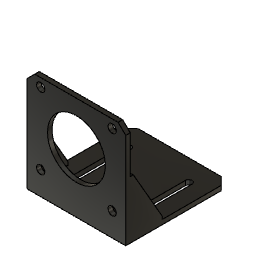
NEMA23 bracket (Autodesk Fusion 360 design; units mm, degrees)
Autodesk Fusion 360 part; units mm, degrees
note: some values were not read from the file. Set by a fixed rule: which sketch regions a step uses.
sketch "NEMA23 bracket front" plane through (0, 0, 0) normal (0, 1, 0) x (1, 0, 0)
  line L0 (-32.5, -3) -> (-32.5, -63)
  line L1 (-32.5, 0) -> (-32.5, -3)
  line L2 (32.5, 0) -> (-32.5, 0)
  line L3 (32.5, -63) -> (32.5, -3)
  line L4 (-32.5, -3) -> (32.5, -3)
  line L5 (-27.5, -68) -> (27.5, -68)
  line L6 (23.55, -15.45) -> (-23.55, -15.45) construction
  line L7 (32.5, -3) -> (32.5, 0)
  circle A0 centre (-23.55, -62.55) radius 2.75
  line L8 (32.5, 0) -> (32.5, -68) construction
  line L9 (23.55, -62.55) -> (-23.55, -62.55) construction
  circle A1 centre (23.55, -15.45) radius 2.75
  line L10 (32.5, -3) -> (-32.5, -3)
  circle A2 centre (0, -39) radius 19.05
  line L11 (-23.55, -62.55) -> (-23.55, -15.45) construction
  line L12 (23.55, -15.45) -> (23.55, -62.55) construction
  circle A3 centre (-23.55, -15.45) radius 2.75
  circle A4 centre (23.55, -62.55) radius 2.75
  line L13 (-32.5, -63) -> (-27.5, -68)
  line L14 (27.5, -68) -> (32.5, -63)
  dimension "d22" = 38.1
  dimension "d23" = 39
  dimension "d24" = 5.5
  dimension "d27" = 47.1
  dimension "d28" = 47.1
  dimension "d29" = 47.1
  dimension "d30" = 5.5
  dimension "d31" = 5.5
  dimension "d32" = 5.5
  dimension "d33" = 68
  dimension "d34" = 32.5
  dimension "d35" = 65
  dimension "d36" = 3
  dimension "d37" = 65
  dimension "d39" = 5.45
  dimension "d46" = 5
  dimension "d47" = 5
  constraint coincident L6.start A1.centre
  constraint perpendicular L6 L12
  constraint perpendicular L9 L12
  constraint coincident L9.start L12.end
  constraint coincident A0.centre L9.end
  constraint coincident L6.end L11.end
  constraint coincident L8 L3.start
  measures "d22" diameter of A2
  measures "d23" distance of A2.centre origin
  measures "d24" diameter of A1
  measures "d27" distance of L6.end L6.start
  measures "d28" distance of L6.start L9.start
  measures "d29" distance of A0.centre L9.start
  measures "d30" diameter of A4
  measures "d31" diameter of A0
  measures "d32" diameter of A3
  measures "d33" distance of L2.start L8.end
  measures "d34" distance of L2.start origin
  measures "d35" distance of L1.start L2.start
  measures "d36" distance of L2.start L3.end
  measures "d37" distance of L3.end L0.start
  measures "d39" distance of L9.start L5
  measures "d46" distance of L8.end L5.end
  measures "d47" distance of L8.end L3.start
extrude "Extrude1" add sketch "NEMA23 bracket front" along normal blind 68 contours L1 L2 L4 L7 L10 makes body 1
extrude "Extrude2" add sketch "NEMA23 bracket front" along normal blind 3 contours L0 L3 L4 L5 L10 L13 L14 bodies 1
sketch "NEMA23 bracket side" plane through (0, 0, 0) normal (1, 0, 0) x (0, 1, 0)
  line L0 (3, 3) -> (24, 3)
  line L1 (24, 3) -> (24, 5)
  line L2 (24, 5) -> (5, 38)
  line L3 (5, 38) -> (3, 38)
  line L4 (3, 38) -> (3, 3)
  dimension "d52" = 21
  dimension "d53" = 35
  dimension "d54" = 2
  dimension "d55" = 2
  dimension "d56" = 3
  dimension "d57" = 3
  constraint horizontal L0
  constraint perpendicular L0 L1
  constraint perpendicular L1 L3
  constraint perpendicular L0 L4
  measures "d52" distance of L0.start L0.end
  measures "d53" distance of L0.start L3.end
  measures "d54" distance of L2.end L3.end
  measures "d55" distance of L0.end L1.end
  measures "d56" horizontal distance of origin L0.start
  measures "d57" vertical distance of origin L0.start
extrude "Extrude3" add sketch "NEMA23 bracket side" along normal mid plane 65 bodies 1
extrude "Extrude4" cut sketch "NEMA23 bracket side" along normal mid plane 59 bodies 1
sketch "NEMA23 bracket top" plane through (0, 0, 3) normal (0, 0, 1) x (-1, 0, 0)
  line L0 (32.5, -24) -> (29.5, -24)
  line L1 (29.5, -24) -> (29.5, -3)
  line L2 (29.5, -3) -> (-29.5, -3)
  line L3 (-29.5, -3) -> (-29.5, -24)
  line L4 (-29.5, -24) -> (-32.5, -24)
  line L5 (-32.5, -24) -> (-32.5, -68)
  line L6 (-32.5, -68) -> (32.5, -68)
  line L7 (32.5, -68) -> (32.5, -24)
  line L8 (20, -54) -> (-20, -54) construction
  line L9 (-20, -54) -> (-20, -13) construction
  line L10 (-20, -13) -> (20, -13) construction
  line L11 (20, -13) -> (20, -54) construction
  line L12 (32.5, -68) -> (27.5, -68)
  line L13 (32.5, -68) -> (32.5, -63)
  line L14 (27.5, -68) -> (32.5, -63)
  line L15 (-32.5, -68) -> (-27.5, -68)
  line L16 (-32.5, -68) -> (-32.5, -63)
  line L17 (-32.5, -63) -> (-27.5, -68)
  line L18 (22.15, -54) -> (22.15, -13)
  line L19 (17.85, -54) -> (17.85, -13)
  line L20 (-17.85, -54) -> (-17.85, -13)
  line L21 (-22.15, -54) -> (-22.15, -13)
  arc A0 (17.85, -54) -> (22.15, -54) centre (20, -54) ccw
  arc A1 (22.15, -13) -> (17.85, -13) centre (20, -13) ccw
  arc A2 (-17.85, -13) -> (-22.15, -13) centre (-20, -13) ccw
  arc A3 (-22.15, -54) -> (-17.85, -54) centre (-20, -54) ccw
  dimension "d62" = 40
  dimension "d63" = 41
  dimension "d64" = 13
  dimension "d65" = 4.3
  dimension "d66" = 4.3
  dimension "d67" = 4.3
  dimension "d68" = 4.3
  dimension "d69" = 5
  dimension "d70" = 5
  dimension "d71" = 5
  dimension "d72" = 5
  constraint horizontal L8
  constraint vertical L9
  constraint horizontal L10
  constraint vertical L11
  constraint coincident L8.start L11.end
  constraint coincident L8.end L9.start
  constraint coincident L10.end L11.start
  constraint coincident L9.end L10.start
  constraint coincident L6.end L7.start
  constraint perpendicular L7 L12
  constraint coincident L7 L13.end
  constraint coincident L5.end L6.start
  constraint coincident L6 L15.end
  constraint perpendicular L15 L16
  constraint tangent L18 A1
  constraint parallel L11 L18
  constraint coincident L8 L19.start
  constraint coincident L10 L19.end
  constraint coincident L8 L20.start
  constraint coincident L10 L20.end
  constraint tangent L21 A2
  constraint parallel L9 L21
  measures "d62" distance of L9 L11
  measures "d63" distance of L8 L10
  measures "d64" distance of origin L10
  measures "d65" diameter of A0
  measures "d66" diameter of A3
  measures "d67" diameter of A1
  measures "d68" diameter of A2
  measures "d69" distance of L6.end L12.end
  measures "d70" distance of L6.end L13.end
  measures "d71" distance of L5.end L15.end
  measures "d72" distance of L5.end L16.end
extrude "Extrude5" cut sketch "NEMA23 bracket top" against normal blind 5 contours L18 L19 A0 A1 | L20 L21 A2 A3 bodies 1
extrude "Extrude6" cut sketch "NEMA23 bracket top" against normal blind 5 contours L6 L7 L12 L13 L14 | L5 L6 L15 L16 L17 bodies 1
copy_body "Body->Comp1" bodies 1 removing the originals makes body 2 in component "NEMA23 bracket"
component "NEMA23 bracket" placed x (1, 0, 0) y (0, 1, 0) z (0, 0, 1) at (0, 0, 0)
named bodies: "NEMA23 bracket"
